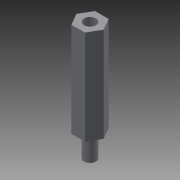
# Autodesk Inventor part: Hex_Standoff
Saved by Autodesk Inventor 2015 SP1 (Build 190203100, 203)
## iProperties
Created: 2016-04-07
Part Number: Hex_Standoff
Material: Generic
Document SubType Name: Modeling
Designer: Ethan
Density: 1 g/cm^3
Appearance: Default
Author: Ethan
Autodesk Inventor part; units mm, degrees
ref_plane "YZ Plane" through (0, 0, 0) normal (1, 0, 0) x (0, 1, 0)
ref_plane "XZ Plane" through (0, 0, 0) normal (0, 1, 0) x (-1, 0, 0)
ref_plane "XY Plane" through (0, 0, 0) normal (0, 0, 1) x (1, 0, 0)
sketch "Sketch1" plane through (0, 0, 0) normal (0, 1, 0) x (-1, 0, 0)
  line L0 (3.6662, 0) -> (1.8331, -3.175)
  line L1 (1.8331, -3.175) -> (-1.8331, -3.175)
  line L2 (-1.8331, -3.175) -> (-3.6662, 0)
  line L3 (-3.6662, 0) -> (-1.8331, 3.175)
  line L4 (-1.8331, 3.175) -> (1.8331, 3.175)
  line L5 (1.8331, 3.175) -> (3.6662, 0)
  circle A0 centre (0, 0) radius 1.5875
  dimension "d0" = 6.35
  dimension "d1" = 3.175
  constraints: 12 end point, 2 coincident, 1 centre point, 13 other
  measures "d0" distance between parallel lines of L3 L0
  measures "d1" diameter of A0
extrude "Extrusion1" add sketch "Sketch1" along normal blind 25.4 contours L0 L1 L2 L3 L4 L5 | A0
extrude "Extrusion2" add sketch "Sketch1" against normal blind 6.35 contours A0
sketch "Sketch2" plane through (0, 25.4, 0) normal (0, 1, 0) x (1, 0, 0)
  circle A0 centre (0, 0) radius 1.5875 projected
extrude "Extrusion3" cut sketch "Sketch2" against normal blind 6.35
body "Solid1"
